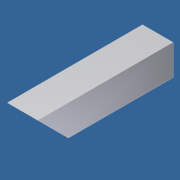
# Autodesk Inventor part: GE-12026-03
Saved by Autodesk Inventor 2012 (Build 160160000, 160)
## iProperties
Created: 2011-07-18
Part Number: GE-12026-03
Document SubType Name: Modeling
Designer: dfoster
Density: 1 g/cm^3
Description: Top Rail Mount
Material: Default
Title: Top Rail Mount
Author: dfoster
Autodesk Inventor part; units mm, degrees
ref_plane "YZ Plane" through (0, 0, 0) normal (1, 0, 0) x (0, 1, 0)
ref_plane "XZ Plane" through (0, 0, 0) normal (0, 1, 0) x (-1, 0, 0)
ref_plane "XY Plane" through (0, 0, 0) normal (0, 0, 1) x (1, 0, 0)
sketch "Sketch1" plane through (0, 0, 0) normal (0, 0, 1) x (1, 0, 0)
  line L0 (0, 0) -> (44.45, 0)
  line L1 (44.45, 0) -> (44.45, 44.45)
  line L2 (44.45, 44.45) -> (0, 44.45)
  line L3 (0, 44.45) -> (0, 0)
  line L4 (3.175, 41.275) -> (41.275, 41.275)
  line L5 (41.275, 41.275) -> (41.275, 3.175)
  line L6 (41.275, 3.175) -> (3.175, 3.175)
  line L7 (3.175, 3.175) -> (3.175, 41.275)
  dimension "d0" = 3.175
  dimension "d1" = 44.45
  constraints: 16 end point, 4 parallel, 3 perpendicular, 1 horizontal, 3 other
  measures "d0" distance between parallel lines of L4 L2
  measures "d1" distance of L1.end L2.end
extrude "Extrusion1" add sketch "Sketch1" along normal blind 196.85
draft "FaceDraft1" angle 45 pull direction (0, -1, 0) faces at (1.0583, 28.575, 196.85) fixed edges at (22.225, 44.45, 196.85)
body "Solid1"
